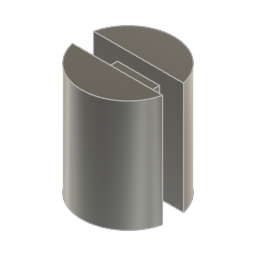
LED spacer v2 (Autodesk Fusion 360 design; units mm, degrees)
Autodesk Fusion 360 part; units mm, degrees
sketch "Sketch1" plane through (0, 0, 0) normal (0, 0, 1) x (1, 0, 0)
  line L0 (-1.6325, 0.381) -> (1.6325, 0.381)
  line L1 (-1.6325, -0.381) -> (1.6325, -0.381)
  line L2 (-0.762, 0) -> (0.762, 0) construction
  line L3 (0, 1.6764) -> (0, -1.6764) construction
  line L4 (-0.762, 0.381) -> (-0.762, -0.381)
  line L5 (0.762, 0.381) -> (0.762, -0.381)
  arc A0 (1.6325, 0.381) -> (-1.6325, 0.381) centre (0, 0) ccw
  arc A1 (-1.6325, -0.381) -> (1.6325, -0.381) centre (0, 0) ccw
  dimension "d1" = 3.3528
  dimension "d2" = 0.762
  dimension "d3" = 1.524
  constraint coincident A0.centre A1.centre
  constraint horizontal L0
  constraint coincident L1.start A0
  constraint parallel L0 L1
  constraint horizontal L2
  constraint coincident A0.centre L2
  constraint symmetric L0 L1 L2
  constraint coincident L3.start A0
  constraint coincident L3.end A0
  constraint perpendicular L2 L3
  constraint coincident A0.centre L3
  constraint coincident L0 L4.start
  constraint coincident L1 L4.end
  constraint perpendicular L1 L4
  constraint coincident L0 L5.start
  constraint coincident L1 L5.end
  constraint perpendicular L1 L5
  constraint concentric A0 A1
  constraint coincident L4 L2.start
  constraint coincident L5 L2.end
  measures "d1" diameter of A0
  measures "d2" distance of L0.start L1.start
  measures "d3" distance of L4.start L5.start
extrude "Extrude1" add sketch "Sketch1" against normal blind 4.064
extrude "Extrude2" cut sketch "Sketch1" against normal blind 0.508 contours L0 L1 L4 L5
